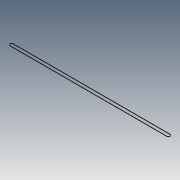
# Autodesk Inventor part: correia-gt2
Saved by Autodesk Inventor 2017 (Build 210142000, 142)
## iProperties
Created: 2018-07-31
Part Number: correia-gt2
Material: Generic
Document SubType Name: Modeling
Designer: Luiz Gustavo
Density: 1 g/cm^3
Appearance: Fine Textured - Black
Author: Luiz Gustavo
Autodesk Inventor part; units mm, degrees
ref_plane "YZ Plane" through (0, 0, 0) normal (1, 0, 0) x (0, 1, 0)
ref_plane "XZ Plane" through (0, 0, 0) normal (0, 1, 0) x (-1, 0, 0)
ref_plane "XY Plane" through (0, 0, 0) normal (0, 0, 1) x (1, 0, 0)
sketch "Sketch1" plane through (0, 0, 0) normal (0, 0, 1) x (1, 0, 0)
  line L0 (-684.25, 0) -> (684.25, 0) construction
  arc A0 (684.25, 12.5) -> (684.25, -12.5) centre (684.25, 0) ccw construction
  arc A1 (-684.25, -12.5) -> (-684.25, 12.5) centre (-684.25, 0) ccw construction
  arc A2 (684.25, 14) -> (684.25, -14) centre (684.25, 0) ccw construction
  arc A3 (-684.25, -14) -> (-684.25, 14) centre (-684.25, 0) ccw construction
  line L1 (684.25, 14) -> (-684.25, 14)
  line L2 (-684.25, 12.5) -> (684.25, 12.5)
  line L3 (684.25, -12.5) -> (-684.25, -12.5)
  line L4 (-684.25, -14) -> (684.25, -14)
  arc A4 (684.25, -14) -> (684.25, 14) centre (684.25, 0) ccw
  arc A5 (684.25, -12.5) -> (684.25, 12.5) centre (684.25, 0) ccw
  arc A6 (-684.25, 14) -> (-684.25, -14) centre (-684.25, 0) ccw
  arc A7 (-684.25, 12.5) -> (-684.25, -12.5) centre (-684.25, 0) ccw
  point P0 (0, 0)
  point P1 (0, 0)
  dimension "d0" = 1368.5
  dimension "d1" = 25
  dimension "d5" = 14
  constraints: 16 point on circle, 10 end point, 8 centre point, 5 coincident, 5 tangent, 4 horizontal, 2 equal radius, 1 midpoint
  measures "d0" distance of L0.start L0.end
  measures "d1" diameter of A0
  measures "d5" radius of A4
extrude "Extrusion1" add sketch "Sketch1" along normal mid plane 6
body "Solid1"
